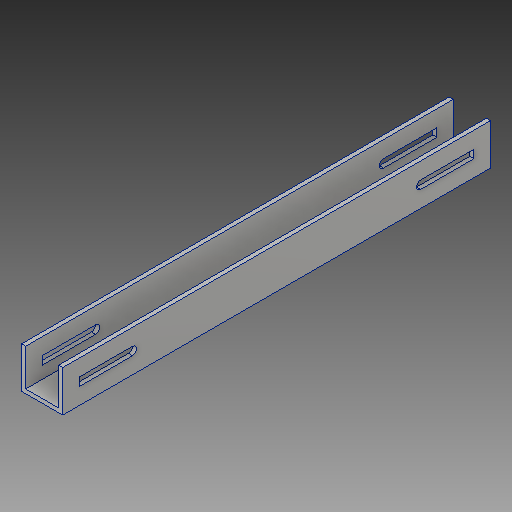
# Autodesk Inventor part: Teemoverthing
Saved by Autodesk Inventor 2017 (Build 210142000, 142)
## iProperties
Created: 2018-01-26
Part Number: Teemoverthing
Material: Aluminum 6061
Document SubType Name: Modeling
Designer: S338674153
Density: 2.7 g/cm^3
Appearance: Aluminum - Flat
Author: S338674153
Autodesk Inventor part; units mm, degrees
ref_plane "YZ Plane" through (0, 0, 0) normal (1, 0, 0) x (0, 1, 0)
ref_plane "XZ Plane" through (0, 0, 0) normal (0, 1, 0) x (-1, 0, 0)
ref_plane "XY Plane" through (0, 0, 0) normal (0, 0, 1) x (1, 0, 0)
sketch "Sketch1" plane through (0, 0, 0) normal (0, 1, 0) x (-1, 0, 0)
  line L0 (0, 0) -> (31.75, 0)
  line L1 (31.75, 0) -> (31.75, -330.2)
  line L2 (31.75, -330.2) -> (0, -330.2)
  line L3 (0, -330.2) -> (0, 0)
  dimension "d0" = 31.75
  dimension "d1" = 330.2
  constraints: 8 end point, 2 parallel, 1 horizontal, 1 perpendicular
  measures "d0" distance of L1.end L2.end
  measures "d1" distance of L0.end L1.end
extrude "Extrusion1" add sketch "Sketch1" along normal blind 3.175
sketch "Sketch8" plane through (0, 3.175, 0) normal (0, 1, 0) x (1, 0, 0)
  line L0 (-31.75, 330.2) -> (-31.75, 0) projected
  line L1 (-31.75, 0) -> (-28.575, 0)
  line L2 (-31.75, 0) -> (0, 0) projected
  line L3 (0, 0) -> (-3.175, 0)
  line L4 (-3.175, 0) -> (-3.175, 330.2)
  line L5 (0, 330.2) -> (-31.75, 330.2) projected
  line L6 (-3.175, 330.2) -> (0, 330.2)
  line L7 (-31.75, 330.2) -> (-28.575, 330.2)
  line L8 (-28.575, 330.2) -> (-28.575, 0)
  line L9 (0, 0) -> (0, 330.2)
  dimension "d41" = 3.175
  dimension "d42" = 3.175
  constraints: 14 end point, 4 point on line, 2 perpendicular, 1 collinear, 1 parallel
  measures "d41" distance of L0.end L1.end
  measures "d42" distance of L2.end L3.end
extrude "Extrusion7" add sketch "Sketch8" along normal blind 28.575 contours L5 L8 L1 L0 | L5 L9 L2 L4
sketch "Sketch10" plane through (0, 0, 0) normal (0, -1, 0) x (1, 0, 0)
  line L0 (0, 0) -> (-31.75, 0) projected
  line L1 (-3.175, -330.2) -> (-28.575, -330.2) projected
  line L2 (0, -330.2) -> (0, 0) projected
  line L3 (-31.75, 0) -> (-31.75, -330.2) projected
  circle A0 centre (-15.875, -162.2821) radius 4.2545
  line L4 (0, -162.2821) -> (-31.75, -162.2821)
  dimension "d60" = 8.509
  constraints: 2 end point, 2 point on line, 1 centre point, 1 midpoint, 1 perpendicular
  measures "d60" diameter of A0
extrude "Extrusion11" cut sketch "Sketch10" against normal through all contours L4 A0 | A0 L4
sketch "Sketch12" plane through (0, 0, 0) normal (1, 0, 0) x (0, 0, -1)
  line L0 (0, 0) -> (0, 31.75) projected
  line L1 (330.2, 3.175) -> (330.2, 31.75) projected
  line L2 (330.2, 31.75) -> (0, 31.75) projected
  line L3 (330.2, 0) -> (0, 0) projected
  line L4 (12.7, 19.05) -> (12.7, 12.7)
  arc A0 (53.975, 12.7) -> (53.975, 19.05) centre (53.975, 15.875) ccw
  line L5 (12.7, 19.05) -> (53.975, 19.05)
  line L6 (12.7, 12.7) -> (53.975, 12.7)
  line L7 (317.5, 19.05) -> (317.5, 12.7)
  arc A1 (276.225, 19.05) -> (276.225, 12.7) centre (276.225, 15.875) ccw
  line L8 (276.225, 19.05) -> (317.5, 19.05)
  line L9 (317.5, 12.7) -> (276.225, 12.7)
  constraints: 12 end point, 4 point on circle, 4 tangent, 2 centre point, 1 horizontal, 1 vertical
extrude "Extrusion13" cut sketch "Sketch12" against normal through all
body "Solid1"
